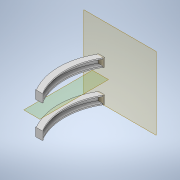
# Autodesk Inventor part: CAMERA_HOLDER
Saved by Autodesk Inventor 2021 (Build 250183000, 183)
## iProperties
Created: 2023-03-21
Part Number: CAMERA_HOLDER
Material: Generic
Document SubType Name: Modeling
Designer: mahmo
Density: 1 g/cm^3
Appearance: Default
Author: mahmo
Autodesk Inventor part; units mm, degrees
ref_plane "YZ Plane" through (0, 0, 0) normal (1, 0, 0) x (0, 1, 0)
ref_plane "XZ Plane" through (0, 0, 0) normal (0, 1, 0) x (-1, 0, 0)
sketch "Sketch1" plane through (0, 0, 0) normal (0, 1, 0) x (-1, 0, 0)
  line L0 (50, 0) -> (43, 0) construction
  line L1 (43, 0) -> (43, -25.5147) construction
  line L2 (43, 0) -> (43, 25.5147) construction
  line L3 (47.5, 26.0147) -> (38.5, 26.0147) construction
  line L4 (38.5, 26.0147) -> (38.5, 25.0147) construction
  line L5 (38.5, 25.0147) -> (47.5, 25.0147) construction
  line L6 (47.5, 25.0147) -> (47.5, 26.0147) construction
  line L7 (47.5, 26.0147) -> (38.5, 25.0147) construction
  line L8 (38.5, 26.0147) -> (47.5, 25.0147) construction
  line L9 (47.5, -25.0147) -> (38.5, -25.0147) construction
  line L10 (38.5, -25.0147) -> (38.5, -26.0147) construction
  line L11 (38.5, -26.0147) -> (47.5, -26.0147) construction
  line L12 (47.5, -26.0147) -> (47.5, -25.0147) construction
  line L13 (47.5, -25.0147) -> (38.5, -26.0147) construction
  line L14 (38.5, -25.0147) -> (47.5, -26.0147) construction
  arc A0 (43.2928, -25.0147) -> (43.2928, 25.0147) centre (0, 0) ccw
  dimension "d1" = 7
  dimension "d2" = 9
  dimension "d3" = 1
  dimension "d4" = 9
  dimension "d5" = 1
  constraints: 30 end point, 4 midpoint, 4 parallel, 3 horizontal, 3 perpendicular, 3 point on circle, 3 point on line, 1 centre point, 1 coincident
  measures "d1" distance of L0.start L0.end
  measures "d2" distance of L5.end L4.end
  measures "d3" distance of L4.end L3.end
  measures "d4" distance of L11.end L10.end
  measures "d5" distance of L10.end L9.end
ref_plane "Work Plane1" through (-43.2928, 0, -25.0147) normal (0, 0, 1) x (1, 0, 0)
sketch "Sketch2" plane through (-43.2928, 0, -25.0147) normal (0, 0, 1) x (1, 0, 0)
  line L0 (4, -2.5) -> (0, -2.5)
  line L1 (0, -2.5) -> (0, -3.5)
  line L2 (0, -3.5) -> (4, -3.5)
  line L3 (4, -3.5) -> (4, -2.5)
  line L4 (4, 2.5) -> (0, 2.5)
  line L5 (0, 3.5) -> (4, 3.5)
  line L6 (4, 3.5) -> (4, 2.5)
  line L7 (-1, 3.5) -> (-1, -3.5)
  line L8 (-1, -3.5) -> (0, -3.5)
  line L9 (0, -3.5) -> (0, 3.5)
  line L10 (-0.9062, 0) -> (-1.9062, 0) construction
  line L11 (-1, 3.5) -> (0, 3.5)
  point P0 (43.2928, 0)
  point P1 (0, 0)
  point P2 (0, -3.5)
  point P3 (0, -2.5)
  point P4 (0, 2.5)
  constraints: 24 end point, 4 parallel, 2 horizontal, 1 collinear, 1 perpendicular
sweep "Sweep1" add profiles "Sketch2" path "Sketch1" keep normal constant yes
sketch "Sketch3" plane through (-44.2928, -3.5, 25.0147) normal (0, 0, 1) x (1, 0, 0)
  line L0 (0, 0) -> (5, 0) projected
  line L1 (5, 0) -> (5, 1) projected
  line L2 (5, 1) -> (1, 1) projected
  line L3 (1, 1) -> (1, 6) projected
  line L4 (1, 6) -> (5, 6) projected
  line L5 (5, 6) -> (5, 7) projected
  line L6 (5, 7) -> (0, 7) projected
  line L7 (0, 7) -> (0, 0) projected
  line L8 (5, 7) -> (0, 7) projected
  line L9 (5, 7) -> (5.5, 7)
  line L10 (5.5, 7) -> (5.5, 0)
  line L11 (5.5, 0) -> (5, 0)
  point P0 (44.2928, 3.5)
  dimension "d16" = 0.5
  constraints: 6 end point, 2 perpendicular, 1 point on line
  measures "d16" distance of L5.end L9.end
extrude "Extrusion1" add sketch "Sketch3" along normal blind 1
mirror "Mirror1" about plane through (0, 0, 0) normal (0, 0, 1) of "Extrusion1"
ref_plane "Work Plane2" through (-44.2928, -13.5, 26.0147) normal (0, -1, 0) x (1, 0, 0)
mirror "Mirror2" about plane through (-44.2928, -13.5, 26.0147) normal (0, -1, 0)
body "Solid1"
